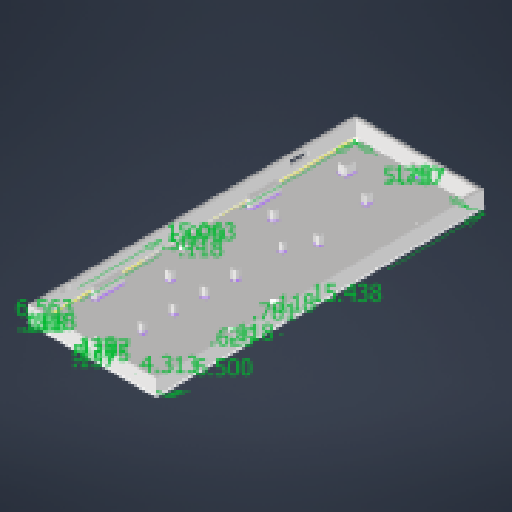
# Autodesk Inventor part: bottom_case
Saved by Autodesk Inventor 2026.2 (Build 302298010, 298A)
## iProperties
Created: 2026-04-02
Part Number: bottom_case
Material: Generic
Document SubType Name: Modeling
Designer: Bradley
Density: 1 g/cm^3
Appearance: Default
Author: Bradley
Autodesk Inventor part; units mm, degrees
ref_plane "YZ Plane" through (0, 0, 0) normal (1, 0, 0) x (0, 1, 0)
ref_plane "XZ Plane" through (0, 0, 0) normal (0, 1, 0) x (-1, 0, 0)
ref_plane "XY Plane" through (0, 0, 0) normal (0, 0, 1) x (1, 0, 0)
sketch "Sketch1" plane through (0, 0, 0) normal (0, 1, 0) x (-1, 0, 0)
  line L0 (0, 0) -> (0, -392.113)
  line L1 (0, -392.113) -> (146.05, -392.113)
  line L2 (146.05, -392.113) -> (146.05, 0)
  line L3 (146.05, 0) -> (0, 0)
  line L4 (148.05, 2) -> (148.05, -394.113)
  line L5 (148.05, -394.113) -> (-2, -394.113)
  line L6 (-2, -394.113) -> (-2, 2)
  line L7 (-2, 2) -> (148.05, 2)
  line L8 (152.05, 6) -> (152.05, -398.113)
  line L9 (152.05, -398.113) -> (-6, -398.113)
  line L10 (-6, -398.113) -> (-6, 6)
  line L11 (-6, 6) -> (152.05, 6)
  dimension "d0" = 146.05
  dimension "d1" = 392.113
  dimension "d2" = 2
  dimension "d3" = 4
  constraints: 24 end point, 3 perpendicular, 2 vertical, 1 horizontal, 6 other
  measures "d0" distance of L0.end L1.end
  measures "d1" distance of L0.start L0.end
  measures "d2" distance between parallel lines of L2 L4
  measures "d3" distance between parallel lines of L7 L11
extrude "Extrusion1" add sketch "Sketch1" along normal blind 2 contours L3 L2 L1 L0
sketch "Sketch2" plane through (0, 2, 0) normal (0, 1, 0) x (1, 0, 0)
  circle A0 centre (-141.287, 4.763) radius 1.5
  line L0 (-146.05, 392.113) -> (-146.05, 0) projected
  line L1 (-146.05, 0) -> (0, 0) projected
  circle A1 centre (-4.762, 4.763) radius 1.5
  circle A2 centre (-141.287, 387.351) radius 1.5
  circle A3 centre (-4.762, 387.351) radius 1.5
  circle A4 centre (-15.875, 109.538) radius 1.5
  circle A5 centre (-19.844, 165.1) radius 1.5
  line L2 (0, 0) -> (0, 392.113) projected
  circle A6 centre (-133.35, 166.688) radius 1.5
  dimension "d6" = 3
  dimension "d7" = 4.763
  dimension "d8" = 4.763
  dimension "d11" = 136.525
  dimension "d14" = 382.588
  dimension "d19" = 3
  dimension "d20" = 3
  dimension "d21" = 109.538
  dimension "d22" = 15.875
  dimension "d23" = 19.844
  dimension "d24" = 165.1
  dimension "d25" = 3
  dimension "d26" = 12.7
  dimension "d27" = 166.688
  constraints: 7 centre point, 1 horizontal, 1 vertical, 6 other
  measures "d6" diameter of A0
  measures "d7" distance from line of L0 A0.centre
  measures "d8" distance from line of L1 A0.centre
  measures "d11" distance of A0.centre A1.centre
  measures "d14" distance of A0.centre A2.centre
  measures "d19" diameter of A4
  measures "d20" diameter of A5
  measures "d21" distance from line of L1 A4.centre
  measures "d22" distance from line of L2 A4.centre
  measures "d23" distance from line of L2 A5.centre
  measures "d24" distance from line of L1 A5.centre
  measures "d25" diameter of A6
  measures "d26" distance from line of L0 A6.centre
  measures "d27" distance from line of L1 A6.centre
extrude "Extrusion2" cut sketch "Sketch2" against normal through all contours A0 | A1 | A2 | A3
extrude "Extrusion3" cut sketch "Sketch2" against normal through all contours A4 | A5 | A6
sketch "Sketch3" plane through (0, 2, 0) normal (0, 1, 0) x (1, 0, 0)
  line L0 (-84.3679, 9) -> (-64.3679, 9)
  line L1 (-64.3679, 9) -> (-64.3679, 12)
  line L2 (-64.3679, 12) -> (-84.3679, 12)
  line L3 (-84.3679, 12) -> (-84.3679, 9)
  line L4 (-146.05, 0) -> (0, 0) projected
  line L5 (-73.7475, 386.8564) -> (-53.7475, 386.8564)
  line L6 (-53.7475, 386.8564) -> (-53.7475, 389.8564)
  line L7 (-53.7475, 389.8564) -> (-73.7475, 389.8564)
  line L8 (-73.7475, 389.8564) -> (-73.7475, 386.8564)
  line L9 (-138.522, 93.7104) -> (-132.6553, 93.7104)
  line L10 (-132.6553, 93.7104) -> (-132.6553, 57.4897)
  line L11 (-132.6553, 57.4897) -> (-138.522, 57.4897)
  line L12 (-138.522, 57.4897) -> (-138.522, 93.7104)
  line L13 (-139.3528, 286.4335) -> (-133.4861, 286.4335)
  line L14 (-133.4861, 286.4335) -> (-133.4861, 250.2128)
  line L15 (-133.4861, 250.2128) -> (-139.3528, 250.2128)
  line L16 (-139.3528, 250.2128) -> (-139.3528, 286.4335)
  line L17 (-72.3966, 93.7104) -> (-67.9097, 93.7104)
  line L18 (-67.9097, 93.7104) -> (-67.9097, 89.2212)
  line L19 (-67.9097, 89.2212) -> (-72.3966, 89.2212)
  line L20 (-72.3966, 89.2212) -> (-72.3966, 93.7104)
  line L21 (-58.1279, 258.8361) -> (-52.0116, 258.8361)
  line L22 (-52.0116, 258.8361) -> (-52.0116, 252.7967)
  line L23 (-52.0116, 252.7967) -> (-58.1279, 252.7967)
  line L24 (-58.1279, 252.7967) -> (-58.1279, 258.8361)
  line L25 (-7.6429, 335.5882) -> (-3.3218, 335.5882)
  line L26 (-3.3218, 335.5882) -> (-3.3218, 328.2515)
  line L27 (-3.3218, 328.2515) -> (-7.6429, 328.2515)
  line L28 (-7.6429, 328.2515) -> (-7.6429, 335.5882)
  line L29 (-119.2414, 356.2386) -> (-109.9087, 356.2386)
  line L30 (-109.9087, 356.2386) -> (-109.9087, 343.6818)
  line L31 (-109.9087, 343.6818) -> (-119.2414, 343.6818)
  line L32 (-119.2414, 343.6818) -> (-119.2414, 356.2386)
  line L33 (-71.9772, 55.173) -> (-67.3534, 55.173)
  line L34 (-67.3534, 55.173) -> (-67.3534, 50.4586)
  line L35 (-67.3534, 50.4586) -> (-71.9772, 50.4586)
  line L36 (-71.9772, 50.4586) -> (-71.9772, 55.173)
  line L37 (-112.3115, 129.4321) -> (-105.8709, 129.4321)
  line L38 (-105.8709, 129.4321) -> (-105.8709, 122.9553)
  line L39 (-105.8709, 122.9553) -> (-112.3115, 122.9553)
  line L40 (-112.3115, 122.9553) -> (-112.3115, 129.4321)
  line L41 (-112.3115, 257.1779) -> (-106.4365, 257.1779)
  line L42 (-106.4365, 257.1779) -> (-106.4365, 251.2133)
  line L43 (-106.4365, 251.2133) -> (-112.3115, 251.2133)
  line L44 (-112.3115, 251.2133) -> (-112.3115, 257.1779)
  line L45 (-71.9772, 131.1422) -> (-66.6479, 131.1422)
  line L46 (-66.6479, 131.1422) -> (-66.6479, 127.27)
  line L47 (-66.6479, 127.27) -> (-71.9772, 127.27)
  line L48 (-71.9772, 127.27) -> (-71.9772, 131.1422)
  line L49 (-71.9772, 170.2584) -> (-66.6479, 170.2584)
  line L50 (-66.6479, 170.2584) -> (-66.6479, 164.8496)
  line L51 (-66.6479, 164.8496) -> (-71.9772, 164.8496)
  line L52 (-71.9772, 164.8496) -> (-71.9772, 170.2584)
  line L53 (-71.9772, 227.794) -> (-67.3534, 227.794)
  line L54 (-67.3534, 227.794) -> (-67.3534, 222.7529)
  line L55 (-67.3534, 222.7529) -> (-71.9772, 222.7529)
  line L56 (-71.9772, 222.7529) -> (-71.9772, 227.794)
  line L57 (-71.9772, 333.6214) -> (-66.6479, 333.6214)
  line L58 (-66.6479, 333.6214) -> (-66.6479, 325.5838)
  line L59 (-66.6479, 325.5838) -> (-71.9772, 325.5838)
  line L60 (-71.9772, 325.5838) -> (-71.9772, 333.6214)
  dimension "d30" = 20
  dimension "d31" = 3
  dimension "d32" = 12
  dimension "d35" = 20
  dimension "d36" = 3
  constraints: 120 end point, 30 parallel, 15 horizontal, 15 perpendicular, 2 point on line
  measures "d30" distance of L2.end L1.end
  measures "d31" distance of L2.end L0.start
  measures "d32" distance between parallel lines of L4 L2
  measures "d35" distance of L7.end L6.end
  measures "d36" distance of L7.end L5.start
extrude "Extrusion4" add sketch "Sketch3" along normal blind 11 contours L3 L2 L1 L0
extrude "Extrusion5" add sketch "Sketch3" along normal blind 11 contours L8 L7 L6 L5 | L9 L10 L11 L12 | L13 L14 L15 L16 | L17 L18 L19 L20 | L21 L22 L23 L24 | L25 L26 L27 L28 | L29 L30 L31 L32 | L33 L34 L35 L36 | L37 L38 L39 L40 | L41 L42 L43 L44 | L45 L46 L47 L48 | L49 L50 L51 L52 | L53 L54 L55 L56 | L57 L58 L59 L60
extrude "Extrusion6" add sketch "Sketch1" along normal blind 20 contours L8 L9 L10 L11
sketch "Sketch4" plane through (-152.05, 0, -398.113) normal (-1, 0, 0) x (0, 0, 1)
  line L0 (358.1458, 18.6338) -> (368.1975, 18.6338)
  line L1 (368.1975, 18.6338) -> (368.1975, 14.8444)
  line L2 (368.1975, 14.8444) -> (358.1458, 14.8444)
  line L3 (358.1458, 14.8444) -> (358.1458, 18.6338)
  point P0 (398.113, 0)
  point P1 (212.9873, 26.1445)
  point P2 (212.9873, 26.1445)
  point P3 (212.9873, 26.1445)
  constraints: 8 end point, 2 coincident, 2 parallel, 1 horizontal, 1 perpendicular
extrude "Extrusion7" cut sketch "Sketch4" against normal blind 20
sketch "Sketch5" plane through (-152.05, 0, -398.113) normal (-1, 0, 0) x (0, 0, 1)
  line L0 (6, 2) -> (398.113, 2) projected
  line L1 (85.2683, 2) -> (62.6972, 2)
  line L2 (62.6972, 15.9667) -> (85.2683, 15.9667)
  line L3 (85.2683, 15.9667) -> (85.2683, 8.6713)
  line L4 (85.2683, 8.6713) -> (62.6972, 8.6713)
  line L5 (62.6972, 8.6713) -> (62.6972, 15.9667)
  point P0 (398.113, 0)
  constraints: 10 end point, 2 parallel, 1 horizontal, 1 perpendicular, 1 point on line
extrude "Extrusion10" cut sketch "Sketch5" against normal blind 20
body "Solid1"
